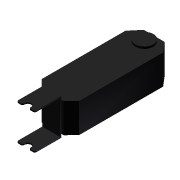
# Autodesk Inventor part: ForeArm
Saved by Autodesk Inventor 2012 (Build 160160000, 160)
## iProperties
Created: 2013-02-21
Part Number: ForeArm
Material: Default
Document SubType Name: Modeling
Designer: Andrew
Density: 1 g/cm^3
Author: Andrew
Autodesk Inventor part; units mm, degrees
ref_plane "YZ Plane" through (0, 0, 0) normal (1, 0, 0) x (0, 1, 0)
ref_plane "XZ Plane" through (0, 0, 0) normal (0, 1, 0) x (-1, 0, 0)
ref_plane "XY Plane" through (0, 0, 0) normal (0, 0, 1) x (1, 0, 0)
sketch "Sketch1" plane through (0, 0, 0) normal (0, 0, 1) x (1, 0, 0)
  line L0 (22.975, -85.9934) -> (22.975, 16.5133)
  line L1 (22.975, 16.5133) -> (13.1755, 28.0421)
  arc A0 (13.1755, 28.0421) -> (12.4, 28.6015) centre (11.6516, 26.7468) ccw
  arc A1 (-12.4, 28.6015) -> (-13.1755, 28.0421) centre (-11.6516, 26.7468) ccw
  line L2 (-13.1755, 28.0421) -> (-22.975, 16.5133)
  line L3 (-22.975, 16.5133) -> (-22.975, -85.4265)
  line L4 (-12.975, -95.4265) -> (-22.975, -85.4265)
  line L5 (-12.975, -95.4265) -> (13.594, -95.4265)
  line L6 (22.975, -85.9934) -> (13.594, -95.4265)
  line L7 (-6, -127.9265) -> (-8.9861, -127.9265)
  arc A2 (-6, -127.9265) -> (-4, -125.9265) centre (-6, -125.9265) ccw
  line L8 (-4, -125.9265) -> (-4, -125.4265)
  arc A3 (4, -125.4265) -> (-4, -125.4265) centre (0, -125.4265) ccw
  line L9 (4, -125.9265) -> (4, -125.4265)
  arc A4 (4, -125.9265) -> (6, -127.9265) centre (6, -125.9265) ccw
  line L10 (8.9861, -127.9265) -> (6, -127.9265)
  arc A5 (8.9861, -127.9265) -> (10.983, -126.0376) centre (8.9861, -125.9265) ccw
  arc A6 (10.983, -126.0376) -> (11, -125.4265) centre (0, -125.4265) ccw
  line L11 (11, -125.4265) -> (11, -96.9265)
  line L12 (-11, -125.4265) -> (-11, -96.9265)
  arc A7 (-11, -125.4265) -> (-10.983, -126.0376) centre (0, -125.4265) ccw
  arc A8 (-10.983, -126.0376) -> (-8.9861, -127.9265) centre (-8.9861, -125.9265) ccw
  line L13 (-11, -96.9265) -> (-11, -95.4265)
  line L14 (11, -96.9265) -> (11, -95.4265)
  line L15 (-12.4, 28.6015) -> (12.4, 28.6015)
  circle A9 centre (0, 16.6015) radius 11
  dimension "d0" = 22
  constraints: 6 end point, 3 perpendicular, 2 point on line, 1 centre point, 1 coincident
  measures "d0" diameter of A9
extrude "Extrusion1" add sketch "Sketch1" along normal mid plane 36 contours L6 L5 L4 L3 L2 A1 L15 A0 L1 L0
extrude "Extrusion2" add sketch "Sketch1" along normal mid plane 41 contours A9
sketch "Sketch2" plane through (-12.975, -95.4265, 18) normal (0, -1, 0) x (1, 0, 0)
  line L0 (1.975, 4) -> (23.975, 4)
  line L1 (23.975, 4) -> (23.975, -40)
  line L2 (23.975, -40) -> (1.975, -40)
  line L3 (1.975, -40) -> (1.975, 4)
  point P0 (12.975, -18)
  point P1 (12.975, -18)
  point P2 (12.975, -18)
  dimension "d5" = 22
  dimension "d6" = 44
  dimension "d16" = 22
  constraints: 8 end point, 2 parallel, 1 coincident, 1 horizontal, 1 perpendicular
  measures "d5" distance of L1.end L2.end
  measures "d6" distance of L0.end L1.end
  measures "d16" distance from line of point (12.975, -18) L2
extrude "Extrusion3" add sketch "Sketch2" along normal blind 1.5
sketch "Sketch3" plane through (-12.975, -96.9265, 18) normal (0, -1, 0) x (1, 0, 0)
  line L0 (23.975, 4) -> (23.975, -40) projected
  line L1 (1.975, -40) -> (1.975, 4) projected
  line L2 (1.975, 4) -> (23.975, 4)
  line L3 (23.975, 4) -> (23.975, 2.5)
  line L4 (23.975, 2.5) -> (1.975, 2.5)
  line L5 (1.975, 2.5) -> (1.975, 4)
  line L6 (23.975, -40) -> (1.975, -40)
  line L7 (1.975, -40) -> (1.975, -38.5)
  line L8 (1.975, -38.5) -> (23.975, -38.5)
  line L9 (23.975, -38.5) -> (23.975, -40)
  point P0 (12.975, -18)
  dimension "d9" = 1.5
  dimension "d10" = 1.5
  constraints: 16 end point, 4 parallel, 2 horizontal, 2 perpendicular, 2 point on line
  measures "d9" distance of L2.end L3.end
  measures "d10" distance of L6.end L7.end
extrude "Extrusion4" add sketch "Sketch3" along normal blind 32 contours L0 L4 L1 L2 | L0 L6 L1 L8
sketch "Sketch4" plane through (11, -95.4265, -22) normal (0, 0, -1) x (-1, 0, 0)
  line L0 (22, 0) -> (22, -33.5) projected
  line L1 (0, 0) -> (22, 0) projected
  line L2 (0, 0) -> (0, -33.5) projected
  line L3 (0, -33.5) -> (22, -33.5) projected
  arc A0 (15, -30) -> (7, -30) centre (11, -30) ccw projected
  arc A1 (5, -32.5) -> (7, -30.5) centre (5, -30.5) ccw projected
  line L4 (2.0139, -32.5) -> (5, -32.5) projected
  line L5 (15, -30.5) -> (15, -30) projected
  line L6 (7, -30.5) -> (7, -30) projected
  arc A2 (0.017, -30.6111) -> (2.0139, -32.5) centre (2.0139, -30.5) ccw projected
  line L7 (17, -32.5) -> (19.9861, -32.5) projected
  arc A3 (15, -30.5) -> (17, -32.5) centre (17, -30.5) ccw projected
  arc A4 (19.9861, -32.5) -> (21.983, -30.6111) centre (19.9861, -30.5) ccw projected
  arc A5 (21.983, -30.6111) -> (22, -30) centre (11, -30) ccw projected
  arc A6 (0, -30) -> (0.017, -30.6111) centre (11, -30) ccw projected
  point P0 (11, 95.4265)
extrude "Extrusion5" cut sketch "Sketch4" against normal through all contours L0 L3 L2 A6 A2 L4 A1 L6 A0 L5 A3 L7 A4 A5
body "Solid1"
